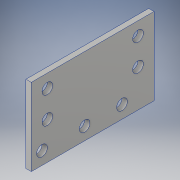
# Autodesk Inventor part: Motorhalterung_Stützleiste
Saved by Autodesk Inventor 2018 (Build 220112000, 112)
## iProperties
Created: 2018-03-26
Part Number: Motorhalterung_Stützleiste
Material: Aluminium 6061
Document SubType Name: Modeling
Designer: Julian
Density: 2.7 g/cm^3
Appearance: Aluminium - flach
Author: Julian
Autodesk Inventor part; units mm, degrees
ref_plane "YZ Plane" through (0, 0, 0) normal (1, 0, 0) x (0, 1, 0)
ref_plane "XZ Plane" through (0, 0, 0) normal (0, 1, 0) x (-1, 0, 0)
ref_plane "XY Plane" through (0, 0, 0) normal (0, 0, 1) x (1, 0, 0)
sketch "Skizze1" plane through (0, 0, 0) normal (1, 0, 0) x (0, 1, 0)
  line L0 (0, 0) -> (115, 0)
  line L1 (115, 0) -> (115, -72.5)
  line L2 (115, -72.5) -> (0, -72.5)
  line L3 (0, -72.5) -> (0, 0)
  line L4 (115, 0) -> (115, -25)
  line L5 (115, -25) -> (100, -25)
  line L6 (100, -25) -> (100, -12.5)
  line L7 (100, -12.5) -> (100, -25)
  line L8 (100, -25) -> (100, -37.5)
  line L9 (100, -25) -> (15, -25)
  line L10 (15, -25) -> (15, -12.5)
  line L11 (15, -12.5) -> (15, -25)
  line L12 (15, -25) -> (15, -37.5)
  circle A0 centre (100, -12.5) radius 5
  circle A1 centre (100, -37.5) radius 5
  circle A2 centre (15, -12.5) radius 5
  circle A3 centre (15, -37.5) radius 5
  line L13 (115, -72.5) -> (85, -72.5)
  line L14 (85, -72.5) -> (50, -72.5)
  line L15 (50, -72.5) -> (10, -72.5)
  line L16 (10, -72.5) -> (10, -60.5)
  line L17 (50, -72.5) -> (50, -60.5)
  line L18 (85, -72.5) -> (85, -60.5)
  circle A4 centre (85, -60.5) radius 5
  circle A5 centre (50, -60.5) radius 5
  circle A6 centre (10, -60.5) radius 5
  dimension "d0" = 115
  dimension "d1" = 72.5
  dimension "d2" = 25
  dimension "d3" = 15
  dimension "d4" = 12.5
  dimension "d5" = 85
  dimension "d6" = 10
  dimension "d7" = 10
  dimension "d8" = 10
  dimension "d9" = 10
  dimension "d10" = 30
  dimension "d11" = 35
  dimension "d12" = 40
  dimension "d13" = 12
  dimension "d14" = 12
  dimension "d15" = 12
  dimension "d16" = 10
  dimension "d17" = 10
  dimension "d18" = 10
  constraints: 38 end point, 7 centre point, 7 coincident, 6 perpendicular, 6 point on line, 4 equal length, 2 horizontal, 1 vertical
  measures "d0" distance of L1.end L2.end
  measures "d1" distance between parallel lines of L2 L0
  measures "d2" distance of L0.end L4.end
  measures "d3" distance of L4.end L5.end
  measures "d4" distance of L5.end L8.end
  measures "d5" distance of L5.end L9.end
  measures "d6" diameter of A0
  measures "d7" diameter of A1
  measures "d8" diameter of A2
  measures "d9" diameter of A3
  measures "d10" distance of L1.end L13.end
  measures "d11" distance of L13.end L14.end
  measures "d12" distance of L14.end L15.end
  measures "d13" distance of L15.end L16.end
  measures "d14" distance of L14.end L17.end
  measures "d15" distance of L13.end L18.end
  measures "d16" diameter of A4
  measures "d17" diameter of A5
  measures "d18" diameter of A6
extrude "Extrusion1" add sketch "Skizze1" along normal blind 5
